Autodesk Fusion 360 part; units mm, degrees
note: some values were not read from the file. Set by a fixed rule: which face or edge a step refers to.
(part 2 of 2)
sketch "Skizze2" plane through (0, 10, 0) normal (0, 1, 0) x (-1, 0, 0)
  line L0 (40, -40) -> (45, -40)
  line L1 (45, -40) -> (45, 40)
  line L2 (45, 40) -> (40, 40)
  line L3 (40, 40) -> (40, 45)
  line L4 (40, 45) -> (-40, 45)
  line L5 (-40, 45) -> (-40, 40)
  line L6 (-40, 40) -> (-45, 40)
  line L7 (-45, 40) -> (-45, -40)
  line L8 (-45, -40) -> (-40, -40)
  line L9 (-40, -40) -> (-40, -45)
  line L10 (-40, -45) -> (40, -45)
  line L11 (40, -45) -> (40, -40)
  line L12 (82.5, 7.5) -> (7.5, 7.5) construction
  line L13 (7.5, 7.5) -> (7.5, 82.5) construction
  line L14 (7.5, 82.5) -> (82.5, 82.5) construction
  line L15 (82.5, 82.5) -> (82.5, 7.5) construction
  line L16 (82.5, 7.5) -> (67.5, 7.5)
  line L17 (67.5, 7.5) -> (67.5, 22.5)
  line L18 (67.5, 22.5) -> (82.5, 22.5)
  line L19 (82.5, 22.5) -> (82.5, 7.5)
  line L20 (7.5, 7.5) -> (22.5, 7.5)
  line L21 (22.5, 7.5) -> (22.5, 22.5)
  line L22 (22.5, 22.5) -> (7.5, 22.5)
  line L23 (7.5, 22.5) -> (7.5, 7.5)
  line L24 (82.5, 82.5) -> (67.5, 82.5)
  line L25 (67.5, 82.5) -> (67.5, 67.5)
  line L26 (67.5, 67.5) -> (82.5, 67.5)
  line L27 (82.5, 67.5) -> (82.5, 82.5)
  line L28 (7.5, 82.5) -> (22.5, 82.5)
  line L29 (22.5, 82.5) -> (22.5, 67.5)
  line L30 (22.5, 67.5) -> (7.5, 67.5)
  line L31 (7.5, 67.5) -> (7.5, 82.5)
  line L32 (75, 67.5) -> (22.5, 15)
  line L33 (15, 22.5) -> (67.5, 75)
  line L34 (75, 22.5) -> (22.5, 75)
  line L35 (67.5, 15) -> (15, 67.5)
  line L36 (45, 7.5) -> (45, 82.5) construction
  line L37 (82.5, 45) -> (7.5, 45) construction
  line L38 (7.5, 7.5) -> (7.5, 82.5) construction
  line L39 (45, 7.5) -> (45, 82.5) construction
  line L40 (67.5, 15) -> (15, 67.5)
  line L41 (67.5, 22.5) -> (82.5, 22.5)
  line L42 (82.5, 22.5) -> (82.5, 7.5)
  line L43 (7.5, 7.5) -> (22.5, 7.5)
  line L44 (7.5, 22.5) -> (7.5, 7.5)
  line L45 (82.5, 82.5) -> (67.5, 82.5)
  line L46 (7.5, 67.5) -> (7.5, 82.5)
  line L47 (22.5, 67.5) -> (7.5, 67.5)
  line L48 (75, 67.5) -> (22.5, 15)
  line L49 (22.5, 82.5) -> (22.5, 67.5)
  line L50 (22.5, 7.5) -> (22.5, 22.5)
  line L51 (67.5, 82.5) -> (67.5, 67.5)
  line L52 (67.5, 67.5) -> (82.5, 67.5)
  line L53 (82.5, 67.5) -> (82.5, 82.5)
  line L54 (22.5, 22.5) -> (7.5, 22.5)
  line L55 (82.5, 45) -> (7.5, 45) construction
  line L56 (67.5, 7.5) -> (67.5, 22.5)
  line L57 (7.5, 82.5) -> (22.5, 82.5)
  line L58 (15, 22.5) -> (67.5, 75)
  line L59 (82.5, 82.5) -> (82.5, 7.5) construction
  line L60 (75, 22.5) -> (22.5, 75)
  line L61 (82.5, 7.5) -> (67.5, 7.5)
  line L62 (7.5, 82.5) -> (82.5, 82.5) construction
  line L63 (82.5, 7.5) -> (7.5, 7.5) construction
  line L64 (-82.5, 7.5) -> (-82.5, 82.5) construction
  line L65 (-45, 7.5) -> (-45, 82.5) construction
  line L66 (-22.5, 15) -> (-75, 67.5)
  line L67 (-22.5, 22.5) -> (-7.5, 22.5)
  line L68 (-7.5, 22.5) -> (-7.5, 7.5)
  line L69 (-82.5, 7.5) -> (-67.5, 7.5)
  line L70 (-82.5, 22.5) -> (-82.5, 7.5)
  line L71 (-7.5, 82.5) -> (-22.5, 82.5)
  line L72 (-82.5, 67.5) -> (-82.5, 82.5)
  line L73 (-67.5, 67.5) -> (-82.5, 67.5)
  line L74 (-15, 67.5) -> (-67.5, 15)
  line L75 (-67.5, 82.5) -> (-67.5, 67.5)
  line L76 (-67.5, 7.5) -> (-67.5, 22.5)
  line L77 (-22.5, 82.5) -> (-22.5, 67.5)
  line L78 (-22.5, 67.5) -> (-7.5, 67.5)
  line L79 (-7.5, 67.5) -> (-7.5, 82.5)
  line L80 (-67.5, 22.5) -> (-82.5, 22.5)
  line L81 (-7.5, 45) -> (-82.5, 45) construction
  line L82 (-22.5, 7.5) -> (-22.5, 22.5)
  line L83 (-82.5, 82.5) -> (-67.5, 82.5)
  line L84 (-75, 22.5) -> (-22.5, 75)
  line L85 (-7.5, 82.5) -> (-7.5, 7.5) construction
  line L86 (-15, 22.5) -> (-67.5, 75)
  line L87 (-7.5, 7.5) -> (-22.5, 7.5)
  line L88 (-82.5, 82.5) -> (-7.5, 82.5) construction
  line L89 (-7.5, 7.5) -> (-82.5, 7.5) construction
  line L90 (-15, -22.5) -> (-67.5, -75)
  line L91 (-82.5, -82.5) -> (-82.5, -7.5) construction
  line L92 (-22.5, -75) -> (-75, -22.5)
  line L93 (-82.5, -22.5) -> (-82.5, -7.5)
  line L94 (-67.5, -7.5) -> (-67.5, -22.5)
  line L95 (-7.5, -45) -> (-82.5, -45) construction
  line L96 (-82.5, -7.5) -> (-67.5, -7.5)
  line L97 (-82.5, -7.5) -> (-67.5, -7.5)
  line L98 (-15, -67.5) -> (-67.5, -15)
  line L99 (-50, -50) -> (-50, -45)
  line L100 (-67.5, -67.5) -> (-82.5, -67.5)
  line L101 (-67.5, -82.5) -> (-67.5, -67.5)
  line L102 (-7.5, -82.5) -> (-22.5, -82.5)
  line L103 (-7.5, -67.5) -> (-7.5, -82.5)
  line L104 (-45, -82.5) -> (-45, -7.5) construction
  line L105 (-67.5, -67.5) -> (-82.5, -67.5)
  line L106 (-67.5, -22.5) -> (-82.5, -22.5)
  line L107 (-7.5, -82.5) -> (-82.5, -82.5) construction
  line L108 (-22.5, -75) -> (-75, -22.5)
  line L109 (-22.5, -67.5) -> (-7.5, -67.5)
  line L110 (-82.5, -22.5) -> (-82.5, -7.5)
  line L111 (-67.5, -7.5) -> (-67.5, -22.5)
  line L112 (-45, -50) -> (-50, -50)
  line L113 (-82.5, -82.5) -> (-67.5, -82.5)
  line L114 (-22.5, -7.5) -> (-22.5, -22.5)
  line L115 (-22.5, -22.5) -> (-7.5, -22.5)
  line L116 (-7.5, -82.5) -> (-82.5, -82.5) construction
  line L117 (-82.5, -82.5) -> (-82.5, -7.5) construction
  line L118 (-82.5, -7.5) -> (-7.5, -7.5) construction
  line L119 (-82.5, -67.5) -> (-82.5, -82.5)
  line L120 (-75, -67.5) -> (-22.5, -15)
  line L121 (-82.5, -7.5) -> (-7.5, -7.5) construction
  line L122 (-15, -22.5) -> (-67.5, -75)
  line L123 (-82.5, -82.5) -> (-67.5, -82.5)
  line L124 (-7.5, -67.5) -> (-7.5, -82.5)
  line L125 (-7.5, -7.5) -> (-22.5, -7.5)
  line L126 (-22.5, -67.5) -> (-7.5, -67.5)
  line L127 (-7.5, -22.5) -> (-7.5, -7.5)
  line L128 (-7.5, -7.5) -> (-7.5, -82.5) construction
  line L129 (-7.5, -82.5) -> (-22.5, -82.5)
  line L130 (-22.5, -22.5) -> (-7.5, -22.5)
  line L131 (-22.5, -82.5) -> (-22.5, -67.5)
  line L132 (-67.5, -22.5) -> (-82.5, -22.5)
  line L133 (-7.5, -45) -> (-82.5, -45) construction
  line L134 (-82.5, -67.5) -> (-82.5, -82.5)
  line L135 (-75, -67.5) -> (-22.5, -15)
  line L136 (-67.5, -82.5) -> (-67.5, -67.5)
  line L137 (-15, -67.5) -> (-67.5, -15)
  line L138 (-45, -82.5) -> (-45, -7.5) construction
  line L139 (-22.5, -82.5) -> (-22.5, -67.5)
  line L140 (-7.5, -7.5) -> (-22.5, -7.5)
  line L141 (-7.5, -7.5) -> (-7.5, -82.5) construction
  line L142 (-7.5, -22.5) -> (-7.5, -7.5)
  line L143 (-22.5, -7.5) -> (-22.5, -22.5)
  line L144 (75, -22.5) -> (22.5, -75)
  line L145 (7.5, -82.5) -> (7.5, -7.5) construction
  line L146 (67.5, -75) -> (15, -22.5)
  line L147 (7.5, -22.5) -> (7.5, -7.5)
  line L148 (22.5, -7.5) -> (22.5, -22.5)
  line L149 (82.5, -45) -> (7.5, -45) construction
  line L150 (7.5, -7.5) -> (22.5, -7.5)
  line L151 (7.5, -7.5) -> (22.5, -7.5)
  line L152 (75, -67.5) -> (22.5, -15)
  line L153 (40, -50) -> (40, -45)
  line L154 (22.5, -67.5) -> (7.5, -67.5)
  line L155 (22.5, -82.5) -> (22.5, -67.5)
  line L156 (82.5, -82.5) -> (67.5, -82.5)
  line L157 (82.5, -67.5) -> (82.5, -82.5)
  line L158 (45, -82.5) -> (45, -7.5) construction
  line L159 (22.5, -67.5) -> (7.5, -67.5)
  line L160 (22.5, -22.5) -> (7.5, -22.5)
  line L161 (82.5, -82.5) -> (7.5, -82.5) construction
  line L162 (67.5, -75) -> (15, -22.5)
  line L163 (67.5, -67.5) -> (82.5, -67.5)
  line L164 (7.5, -22.5) -> (7.5, -7.5)
  line L165 (22.5, -7.5) -> (22.5, -22.5)
  line L166 (45, -50) -> (40, -50)
  line L167 (7.5, -82.5) -> (22.5, -82.5)
  line L168 (67.5, -7.5) -> (67.5, -22.5)
  line L169 (67.5, -22.5) -> (82.5, -22.5)
  line L170 (82.5, -82.5) -> (7.5, -82.5) construction
  line L171 (7.5, -82.5) -> (7.5, -7.5) construction
  line L172 (7.5, -7.5) -> (82.5, -7.5) construction
  line L173 (7.5, -67.5) -> (7.5, -82.5)
  line L174 (15, -67.5) -> (67.5, -15)
  line L175 (7.5, -7.5) -> (82.5, -7.5) construction
  line L176 (75, -22.5) -> (22.5, -75)
  line L177 (7.5, -82.5) -> (22.5, -82.5)
  line L178 (82.5, -67.5) -> (82.5, -82.5)
  line L179 (82.5, -7.5) -> (67.5, -7.5)
  line L180 (67.5, -67.5) -> (82.5, -67.5)
  line L181 (82.5, -22.5) -> (82.5, -7.5)
  line L182 (82.5, -7.5) -> (82.5, -82.5) construction
  line L183 (82.5, -82.5) -> (67.5, -82.5)
  line L184 (67.5, -22.5) -> (82.5, -22.5)
  line L185 (67.5, -82.5) -> (67.5, -67.5)
  line L186 (22.5, -22.5) -> (7.5, -22.5)
  line L187 (82.5, -45) -> (7.5, -45) construction
  line L188 (7.5, -67.5) -> (7.5, -82.5)
  line L189 (15, -67.5) -> (67.5, -15)
  line L190 (22.5, -82.5) -> (22.5, -67.5)
  line L191 (75, -67.5) -> (22.5, -15)
  line L192 (45, -82.5) -> (45, -7.5) construction
  line L193 (67.5, -82.5) -> (67.5, -67.5)
  line L194 (82.5, -7.5) -> (67.5, -7.5)
  line L195 (82.5, -7.5) -> (82.5, -82.5) construction
  line L196 (82.5, -22.5) -> (82.5, -7.5)
  line L197 (67.5, -7.5) -> (67.5, -22.5)
  dimension "d3" = 75
  dimension "d4" = 75
  dimension "d5" = 75
  dimension "d6" = 75
  dimension "d7" = 75
  dimension "d8" = 75
  dimension "d9" = 75
  dimension "d10" = 75
  dimension "d11" = 75
  dimension "d12" = 75
  dimension "d13" = 75
  dimension "d14" = 75
  dimension "d15" = 75
  dimension "d16" = 75
  constraint horizontal L12
  constraint vertical L13
  constraint horizontal L14
  constraint vertical L15
  constraint horizontal L16
  constraint vertical L17
  constraint horizontal L18
  constraint vertical L19
  constraint horizontal L20
  constraint vertical L21
  constraint horizontal L22
  constraint vertical L23
  constraint horizontal L24
  constraint vertical L25
  constraint horizontal L26
  constraint vertical L27
  constraint horizontal L28
  constraint vertical L29
  constraint horizontal L30
  constraint vertical L31
  constraint midpoint L26 L32.start
  constraint midpoint L21 L32.end
  constraint midpoint L22 L33.start
  constraint midpoint L25 L33.end
  constraint midpoint L18 L34.start
  constraint midpoint L29 L34.end
  constraint midpoint L17 L35.start
  constraint midpoint L30 L35.end
  constraint midpoint L12 L36.start
  constraint midpoint L14 L36.end
  constraint midpoint L15 L37.start
  constraint midpoint L13 L37.end
  constraint horizontal L63
  constraint vertical L38
  constraint horizontal L62
  constraint vertical L59
  constraint horizontal L61
  constraint vertical L56
  constraint horizontal L41
  constraint vertical L42
  constraint horizontal L43
  constraint vertical L50
  constraint horizontal L54
  constraint vertical L44
  constraint horizontal L45
  constraint vertical L51
  constraint horizontal L52
  constraint vertical L53
  constraint horizontal L57
  constraint vertical L49
  constraint horizontal L47
  constraint vertical L46
  constraint midpoint L32.start L52
  constraint midpoint L32.end L50
  constraint midpoint L33.start L54
  constraint midpoint L33.end L51
  constraint midpoint L34.start L41
  constraint midpoint L34.end L49
  constraint midpoint L35.start L56
  constraint midpoint L35.end L47
  constraint midpoint L36.start L63
  constraint midpoint L36.end L62
  constraint midpoint L37.start L59
  constraint midpoint L37.end L38
  constraint horizontal L89
  constraint vertical L64
  constraint horizontal L88
  constraint vertical L85
  constraint horizontal L87
  constraint vertical L82
  constraint horizontal L67
  constraint vertical L68
  constraint horizontal L69
  constraint vertical L76
  constraint horizontal L80
  constraint vertical L70
  constraint horizontal L71
  constraint vertical L77
  constraint horizontal L78
  constraint vertical L79
  constraint horizontal L83
  constraint vertical L75
  constraint horizontal L73
  constraint vertical L72
  constraint midpoint L74.start L78
  constraint midpoint L74.end L76
  constraint midpoint L84.start L80
  constraint midpoint L84.end L77
  constraint midpoint L86.start L67
  constraint midpoint L86.end L75
  constraint midpoint L66.start L82
  constraint midpoint L66.end L73
  constraint midpoint L65.start L89
  constraint midpoint L65.end L88
  constraint midpoint L81.start L85
  constraint midpoint L81.end L64
  constraint horizontal L107
  constraint vertical L117
  constraint horizontal L118
  constraint vertical L141
  constraint horizontal L102
  constraint vertical L131
  constraint horizontal L109
  constraint vertical L124
  constraint horizontal L123
  constraint vertical L101
  constraint horizontal L100
  constraint vertical L134
  constraint horizontal L125
  constraint vertical L114
  constraint horizontal L130
  constraint vertical L127
  constraint horizontal L97
  constraint vertical L111
  constraint horizontal L132
  constraint vertical L110
  constraint midpoint L90.start L130
  constraint midpoint L90.end L101
  constraint midpoint L120.start L100
  constraint midpoint L120.end L114
  constraint midpoint L98.start L109
  constraint midpoint L98.end L111
  constraint midpoint L92.start L131
  constraint midpoint L92.end L132
  constraint midpoint L104.start L107
  constraint midpoint L104.end L118
  constraint midpoint L95.start L141
  constraint midpoint L95.end L117
  constraint horizontal L116
  constraint vertical L91
  constraint horizontal L121
  constraint vertical L128
  constraint horizontal L129
  constraint vertical L139
  constraint horizontal L126
  constraint vertical L103
  constraint horizontal L113
  constraint vertical L136
  constraint horizontal L105
  constraint vertical L119
  constraint horizontal L140
  constraint vertical L143
  constraint horizontal L115
  constraint vertical L142
  constraint horizontal L96
  constraint vertical L94
  constraint horizontal L106
  constraint vertical L93
  constraint midpoint L90.start L115
  constraint midpoint L90.end L136
  constraint midpoint L120.start L105
  constraint midpoint L120.end L143
  constraint midpoint L98.start L126
  constraint midpoint L98.end L94
  constraint midpoint L92.start L139
  constraint midpoint L92.end L106
  constraint midpoint L104.start L116
  constraint midpoint L104.end L121
  constraint midpoint L95.start L128
  constraint midpoint L95.end L91
  constraint horizontal L161
  constraint vertical L171
  constraint horizontal L172
  constraint vertical L195
  constraint horizontal L156
  constraint vertical L185
  constraint horizontal L163
  constraint vertical L178
  constraint horizontal L177
  constraint vertical L155
  constraint horizontal L154
  constraint vertical L188
  constraint horizontal L179
  constraint vertical L168
  constraint horizontal L184
  constraint vertical L181
  constraint horizontal L151
  constraint vertical L165
  constraint horizontal L186
  constraint vertical L164
  constraint midpoint L144.start L184
  constraint midpoint L144.end L155
  constraint midpoint L174.start L154
  constraint midpoint L174.end L168
  constraint midpoint L152.start L163
  constraint midpoint L152.end L165
  constraint midpoint L146.start L185
  constraint midpoint L146.end L186
  constraint midpoint L158.start L161
  constraint midpoint L158.end L172
  constraint midpoint L149.start L195
  constraint midpoint L149.end L171
  constraint horizontal L170
  constraint vertical L145
  constraint horizontal L175
  constraint vertical L182
  constraint horizontal L183
  constraint vertical L193
  constraint horizontal L180
  constraint vertical L157
  constraint horizontal L167
  constraint vertical L190
  constraint horizontal L159
  constraint vertical L173
  constraint horizontal L194
  constraint vertical L197
  constraint horizontal L169
  constraint vertical L196
  constraint horizontal L150
  constraint vertical L148
  constraint horizontal L160
  constraint vertical L147
  constraint midpoint L144.start L169
  constraint midpoint L144.end L190
  constraint midpoint L174.start L159
  constraint midpoint L174.end L197
  constraint midpoint L152.start L180
  constraint midpoint L152.end L148
  constraint midpoint L146.start L193
  constraint midpoint L146.end L160
  constraint midpoint L158.start L170
  constraint midpoint L158.end L175
  constraint midpoint L149.start L182
  constraint midpoint L149.end L145
  measures "d3" distance of L12.start L12.end
  measures "d4" distance of L12.start L14.end
  measures "d5" distance of L12.start L12.end
  measures "d6" distance of L12.start L14.end
  measures "d7" distance of L68.end L64.start
  measures "d8" distance of L68.end L71.start
  measures "d9" distance of L102.start L91.start
  measures "d10" distance of L102.start L118.end
  measures "d11" distance of L102.start L91.start
  measures "d12" distance of L102.start L118.end
  measures "d13" distance of L156.start L145.start
  measures "d14" distance of L156.start L172.end
  measures "d15" distance of L156.start L145.start
  measures "d16" distance of L156.start L172.end
ref_plane "Arbeitsebene1" through (75, 15, 75) normal (0, 1, 0) x (-1, 0, 0)
move_body "Verschieben1" [suppressed]
sketch "Skizze3" plane through (0, 15, 0) normal (0, 1, 0) x (1, 0, 0)
hidden bodies 2
